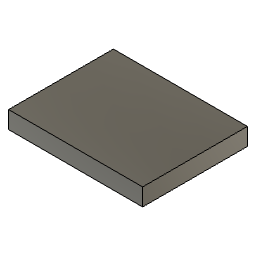
eclipse 2 v21 (Autodesk Fusion 360 archive; units mm, degrees)
design "328 2500mAh battery"
Autodesk Fusion 360 part; units mm, degrees
sketch "Sketch1" plane through (0, 0, 0) normal (0, 0, 1) x (1, 0, 0)
  line L0 (0, 0) -> (61, 0)
  line L1 (61, 0) -> (61, -47.7)
  line L2 (61, -47.7) -> (0, -47.7)
  line L3 (0, -47.7) -> (0, 0)
  dimension "d1" = 61
  dimension "d2" = 47.7
  constraint horizontal L0
  constraint vertical L1
  constraint horizontal L2
  constraint vertical L3
  constraint coincident L0.start L3.end
  measures "d1" distance of L0.start L0.end
  measures "d2" distance of L0.start L2.end
extrude "Extrude1" add sketch "Sketch1" along normal blind 7.9

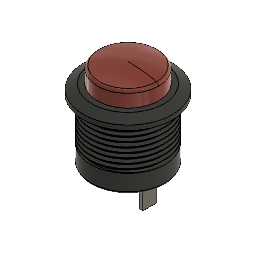
design "1445 16mm button"
Autodesk Fusion 360 part; units mm, degrees
sketch "Sketch1" plane through (0, 0, 0) normal (0, 0, 1) x (1, 0, 0)
  circle A0 centre (0, 0) radius 8.2
  dimension "d1" = 16.4
  measures "d1" diameter of A0
extrude "Extrude1" add sketch "Sketch1" along normal blind 13 makes body 1
sketch "Sketch4" plane through (0, 0, 0) normal (0, 1, 0) x (1, 0, 0)
  line L0 (0, -13) -> (9.5, -13)
  line L1 (9.5, -13) -> (9.5, -14)
  line L2 (0, -13) -> (0, -15)
  line L3 (0, -15) -> (7.6, -15)
  line L4 (-8.2, -13) -> (8.2, -13)
  line L5 (7.6, -15) -> (9.5, -14)
  line L6 (0, -15) -> (0, -19)
  line L7 (6.5, -15) -> (6.5, -18.2)
  spline S0 degree 5 poles (0, -19) (0.2956, -19) (0.8765, -18.9924) (1.7176, -18.9582) (2.7863, -18.8718) (4.0624, -18.7085) (5.0521, -18.5359) (5.7811, -18.3795) (6.2613, -18.262) (6.5, -18.2) knots 0 0 0 0 0 0 0.2 0.4 0.6 0.8 1 1 1 1 1 1
  line L8 (-0.754, -19) -> (0.754, -19)
  line L9 (5.8915, -18.3582) -> (7.1085, -18.0418)
  dimension "d7" = 2
  dimension "d8" = 1
  dimension "d9" = 7.6
  dimension "d10" = 9.5
  dimension "d13" = 4
  dimension "d15" = 3.2
  dimension "d16" = 6.5
  measures "d16" distance of L6 L7
revolve "Revolve1" add sketch "Sketch4" angle 360 about axis through (0, 0, 13) along (0, 0, 1) separate body contours L0 L1 L2 L3 L4 L5 makes body 2
revolve "Revolve2" add sketch "Sketch4" angle 360 about axis through (0, 0, 15) along (0, 0, 1) separate body contours L3 L6 L7 S0 makes body 3
thread "Thread1" "ISO Metric profile 16.0 M16x1 6g" major diameter 15.884 minor diameter 14.741 pitch 1 angle 60 modelled right hand crest width 0.125 on face at (8.1593, -0.8165, 8.6667) from (0, 0, 4) to (0, 0, 13) crest through (7.942, 0, -0.0625) on bodies 1
fillet "Fillet1" radius 0.6 2 edges at (-7.4045, -2.8719, 0) (-6.0601, -2.3505, 18.2) on bodies 1 3
sketch "Sketch6" plane through (0, 0, 0) normal (0, 0, -1) x (1, 0, 0)
  circle A0 centre (0, 0) radius 7.342
  line L0 (3.9, 3) -> (4.66, 3)
  line L1 (4.66, 3) -> (4.66, -3)
  line L2 (4.66, -3) -> (3.9, -3)
  line L3 (3.9, -3) -> (3.9, 3)
  line L4 (3.9, 0) -> (0, 0)
  line L5 (3.9, 1.5) -> (4.66, 1.5)
  line L6 (4.66, 1.5) -> (4.66, -1.5)
  line L7 (4.66, -1.5) -> (3.9, -1.5)
  line L8 (3.9, -1.5) -> (3.9, 1.5)
  dimension "d21" = 0.76
  dimension "d22" = 6
  dimension "d23" = 3.9
  dimension "d24" = 3
  measures "d23" distance of A0.centre
extrude "Extrude2" add sketch "Sketch6" along normal blind 1 separate body contours L0 L1 L3 L5 | L1 L3 L5 L6 L7 L8 | L1 L2 L3 L7 makes body 4
extrude "Extrude3" add sketch "Sketch6" along normal blind 5.5 contours L1 L3 L5 L6 L7 L8 bodies 4
mirror "Mirror1" about plane through (0, 0, 0) normal (1, 0, 0) of bodies 4 makes body 5
equation "d9 = ( 15.2 / 2 ) * 1 mm"
equation "d10 = ( 19 / 2 ) * 1 mm"
equation "d23 = ( 7.8 / 2 ) * 1 mm"
